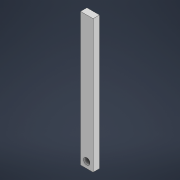
# Autodesk Inventor part: Elbow_Cube_Holder_TestFit_V2
Saved by Autodesk Inventor 2022 (Build 260153000, 153)
## iProperties
Created: 2023-05-10
Part Number: Elbow_Cube_Holder_TestFit_V2
Material: Generic
Document SubType Name: Modeling
Designer: Karl Spiteri
Density: 1 g/cm^3
Appearance: Default
Author: Karl Spiteri
Autodesk Inventor part; units mm, degrees
ref_plane "YZ Plane" through (0, 0, 0) normal (1, 0, 0) x (0, 1, 0)
ref_plane "XZ Plane" through (0, 0, 0) normal (0, 1, 0) x (-1, 0, 0)
ref_plane "XY Plane" through (0, 0, 0) normal (0, 0, 1) x (1, 0, 0)
sketch "Sketch2" plane through (0, 0, 0) normal (0, 0, 1) x (1, 0, 0)
  line L0 (0, 0) -> (-9.9, 0)
  line L1 (-9.9, 0) -> (-9.9, 105)
  line L2 (-9.9, 105) -> (0, 105)
  line L3 (0, 105) -> (0, 0)
  point P0 (-5, 18)
  dimension "d4" = 9.9
  dimension "d5" = 105
  constraints: 8 end point, 2 parallel, 1 horizontal, 1 perpendicular
  measures "d4" distance of L1.end L2.end
  measures "d5" distance of L0.end L1.end
extrude "Extrusion2" add sketch "Sketch2" along normal blind 5
sketch "Sketch3" plane through (0, 0, 5) normal (0, 0, 1) x (1, 0, 0)
  circle A0 centre (-4.95, 5) radius 2.5
  line L0 (-4.95, 7.5) -> (-4.95, 44.5)
  line L1 (-4.95, 7.5) -> (32.05, 7.5) construction
  line L2 (-4.95, 44.5) -> (0, 44.5)
  line L3 (0, 0) -> (0, 105) projected
  line L4 (0, 44.5) -> (-9.9, 44.5)
  line L5 (-9.9, 105) -> (-9.9, 0) projected
  line L6 (-9.9, 44.5) -> (0, 44.5)
  line L7 (0, 44.5) -> (0, 0)
  line L8 (0, 0) -> (-9.9, 0)
  line L9 (-9.9, 0) -> (-9.9, 44.5)
  line L10 (-9.9, 44.5) -> (0, 44.5)
  line L11 (0, 44.5) -> (0, 105)
  line L12 (0, 105) -> (-9.9, 105)
  line L13 (-9.9, 105) -> (-9.9, 44.5)
  line L14 (-4.95, 2.5) -> (-4.95, 0)
  line L15 (-9.9, 0) -> (0, 0) projected
  dimension "d29" = 5
  dimension "d30" = 37
  dimension "d31" = 90
  dimension "d32" = 90
  constraints: 26 end point, 4 parallel, 3 horizontal, 3 perpendicular, 3 point on line, 2 point on circle, 1 centre point, 1 coincident, 1 midpoint, 1 vertical
  measures "d29" diameter of A0
  measures "d30" distance of L0.start L0.end
  measures "d31" angle of L1 L0
  measures "d32" angle of L0 L2
hole "Hole3" at (-4.95, 5, 5) direction (0, 0, -1) diameter 5 depth 6
body "Solid2"
